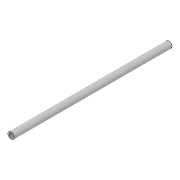
# Autodesk Inventor part: Steel Rod
Saved by Autodesk Inventor 2018.3 (Build 223284000, 284)
## iProperties
Created: 2019-03-08
Part Number: Steel Rod
Material: Generic
Document SubType Name: Modeling
Designer: aye06091
Mass: 0.415739 g
Surface Area: 11.2168 cm^2
Volume: 0.415739 cm^3
Density: 1 g/cm^3
Appearance: Default
Author: aye06091
Autodesk Inventor part; units mm, degrees
ref_plane "YZ Plane" through (0, 0, 0) normal (1, 0, 0) x (0, 1, 0)
ref_plane "XZ Plane" through (0, 0, 0) normal (0, 1, 0) x (-1, 0, 0)
ref_plane "XY Plane" through (0, 0, 0) normal (0, 0, 1) x (1, 0, 0)
sketch "Sketch1" plane through (0, 0, 0) normal (0, 0, 1) x (1, 0, 0)
  circle A0 centre (0, 0) radius 1.5875
  dimension "d0" = 3.175
  constraints: 1 centre point, 1 coincident
  measures "d0" diameter of A0
extrude "Extrusion1" add sketch "Sketch1" along normal blind 76.2
sketch "Sketch2" plane through (0, 0, 76.2) normal (0, 0, 1) x (1, 0, 0)
  circle A0 centre (0, 0) radius 1.5875 projected
  circle A1 centre (0, 0) radius 1.1303
  dimension "d3" = 2.2606
  constraints: 1 centre point, 1 coincident
  measures "d3" diameter of A1
hole "Hole1" at (0, 0, 76.2) direction (0, 0, -1) diameter 2.159 depth 25.4 tip angle 118
sketch "Sketch3" plane through (0, 0, 0) normal (0, 0, -1) x (-1, 0, 0)
  circle A0 centre (0, 0) radius 1.5875 projected
hole "Hole2" at (0, 0, 0) direction (0, 0, 1) diameter 2.159 depth 25.4 tip angle 118
body "Solid1"
